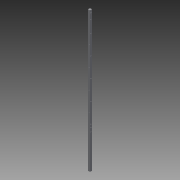
# Autodesk Inventor part: Aluminium Rod
Saved by Autodesk Inventor 2015 (Build 190159000, 159)
## iProperties
Created: 2014-09-22
Part Number: Aluminium Rod
Material: Generic
Document SubType Name: Modeling
Designer: I Rabey
Density: 1 g/cm^3
Appearance: Default
Author: I Rabey
Autodesk Inventor part; units mm, degrees
ref_plane "YZ Plane" through (0, 0, 0) normal (1, 0, 0) x (0, 1, 0)
ref_plane "XZ Plane" through (0, 0, 0) normal (0, 1, 0) x (-1, 0, 0)
ref_plane "XY Plane" through (0, 0, 0) normal (0, 0, 1) x (1, 0, 0)
sketch "Sketch1" plane through (0, 0, 0) normal (0, 1, 0) x (-1, 0, 0)
  line L0 (-6.35, 6.35) -> (6.35, 6.35)
  line L1 (6.35, 6.35) -> (6.35, -6.35)
  line L2 (6.35, -6.35) -> (-6.35, -6.35)
  line L3 (-6.35, -6.35) -> (-6.35, 6.35)
  line L4 (-6.35, 6.35) -> (6.35, -6.35) construction
  line L5 (6.35, 6.35) -> (-6.35, -6.35) construction
  point P0 (0, 0)
  dimension "d0" = 12.7
  dimension "d1" = 12.7
  constraints: 12 end point, 2 midpoint, 2 parallel, 1 horizontal, 1 perpendicular
  measures "d0" distance of L1.end L2.end
  measures "d1" distance of L0.end L1.end
extrude "Extrusion1" add sketch "Sketch1" along normal blind 903
sketch "Sketch3" plane through (6.35, 0, -6.35) normal (1, 0, 0) x (0, 0, -1)
  circle A0 centre (-6.35, 886.5) radius 2.5
  line L0 (-12.7, 903) -> (0, 903) projected
  point P0 (-6.35, 0)
  dimension "d4" = 5
  dimension "d5" = 16.5
  constraints: 1 centre point
  measures "d4" diameter of A0
  measures "d5" distance from line of L0 A0.centre
sketch "Sketch4" plane through (6.35, 0, -6.35) normal (1, 0, 0) x (0, 0, -1)
  circle A0 centre (-6.35, 848.39) radius 2.5
  line L0 (-12.7, 903) -> (0, 903) projected
  point P0 (-6.35, 0)
  dimension "d6" = 5
  dimension "d7" = 54.61
  constraints: 1 centre point
  measures "d6" diameter of A0
  measures "d7" distance from line of L0 A0.centre
sketch "Sketch5" plane through (6.35, 0, -6.35) normal (1, 0, 0) x (0, 0, -1)
  circle A0 centre (-6.35, 772.34) radius 2.5
  line L0 (-12.7, 903) -> (0, 903) projected
  point P0 (-6.35, 0)
  dimension "d8" = 5
  dimension "d9" = 130.66
  constraints: 1 centre point
  measures "d8" diameter of A0
  measures "d9" distance from line of L0 A0.centre
sketch "Sketch6" plane through (6.35, 0, -6.35) normal (1, 0, 0) x (0, 0, -1)
  circle A0 centre (-6.35, 645.34) radius 2.5
  line L0 (-12.7, 903) -> (0, 903) projected
  point P0 (-6.35, 0)
  dimension "d10" = 5
  dimension "d11" = 257.66
  constraints: 1 centre point
  measures "d10" diameter of A0
  measures "d11" distance from line of L0 A0.centre
sketch "Sketch7" plane through (6.35, 0, -6.35) normal (1, 0, 0) x (0, 0, -1)
  circle A0 centre (-6.35, 518.34) radius 2.5
  line L0 (-12.7, 903) -> (0, 903) projected
  point P0 (-6.35, 0)
  dimension "d12" = 5
  dimension "d13" = 384.66
  constraints: 1 centre point
  measures "d12" diameter of A0
  measures "d13" distance from line of L0 A0.centre
sketch "Sketch8" plane through (6.35, 0, -6.35) normal (1, 0, 0) x (0, 0, -1)
  circle A0 centre (-6.35, 391.34) radius 2.5
  line L0 (-12.7, 903) -> (0, 903) projected
  point P0 (-6.35, 0)
  dimension "d14" = 5
  dimension "d15" = 511.66
  constraints: 1 centre point
  measures "d14" diameter of A0
  measures "d15" distance from line of L0 A0.centre
sketch "Sketch9" plane through (6.35, 0, -6.35) normal (1, 0, 0) x (0, 0, -1)
  circle A0 centre (-6.35, 264.34) radius 2.5
  line L0 (-12.7, 903) -> (0, 903) projected
  point P0 (-6.35, 0)
  dimension "d16" = 5
  dimension "d17" = 638.66
  constraints: 1 centre point
  measures "d16" diameter of A0
  measures "d17" distance from line of L0 A0.centre
sketch "Sketch10" plane through (6.35, 0, -6.35) normal (1, 0, 0) x (0, 0, -1)
  circle A0 centre (-6.35, 246.26) radius 2.5
  line L0 (-12.7, 903) -> (0, 903) projected
  point P0 (-6.35, 0)
  dimension "d18" = 5
  dimension "d19" = 656.74
  constraints: 1 centre point
  measures "d18" diameter of A0
  measures "d19" distance from line of L0 A0.centre
sketch "Sketch11" plane through (6.35, 0, -6.35) normal (1, 0, 0) x (0, 0, -1)
  circle A0 centre (-6.35, 220.86) radius 2.5
  line L0 (-12.7, 903) -> (0, 903) projected
  point P0 (-6.35, 0)
  dimension "d20" = 5
  dimension "d21" = 682.14
  constraints: 1 centre point
  measures "d20" diameter of A0
  measures "d21" distance from line of L0 A0.centre
hole "Hole1" at (6.35, 886.5, 0) direction (-1, 0, 0) diameter 5 end through all
hole "Hole2" at (6.35, 848.39, 0) direction (-1, 0, 0) diameter 5 end through all
hole "Hole3" at (6.35, 772.34, 0) direction (-1, 0, 0) diameter 5 end through all
hole "Hole4" at (6.35, 645.34, 0) direction (-1, 0, 0) diameter 5 end through all
hole "Hole5" at (6.35, 518.34, 0) direction (-1, 0, 0) diameter 5 end through all
hole "Hole6" at (6.35, 391.34, 0) direction (-1, 0, 0) diameter 5 end through all
hole "Hole7" at (6.35, 264.34, 0) direction (-1, 0, 0) diameter 5 end through all
hole "Hole8" at (6.35, 246.26, 0) direction (-1, 0, 0) diameter 5 end through all
hole "Hole9" at (6.35, 220.86, 0) direction (-1, 0, 0) diameter 5 end through all
sketch "Sketch21" plane through (6.35, 0, 6.35) normal (0, 0, 1) x (1, 0, 0)
  circle A0 centre (-6.35, 708.84) radius 2.5
  line L0 (-12.7, 903) -> (0, 903) projected
  point P0 (-6.35, 0)
  dimension "d161" = 5
  dimension "d162" = 194.16
  constraints: 1 centre point
  measures "d161" diameter of A0
  measures "d162" distance from line of L0 A0.centre
sketch "Sketch22" plane through (6.35, 0, 6.35) normal (0, 0, 1) x (1, 0, 0)
  circle A0 centre (-6.35, 581.84) radius 2.5
  line L0 (-12.7, 903) -> (0, 903) projected
  point P0 (-6.35, 0)
  dimension "d163" = 5
  dimension "d164" = 321.16
  constraints: 1 centre point
  measures "d163" diameter of A0
  measures "d164" distance from line of A0.centre L0
sketch "Sketch23" plane through (6.35, 0, 6.35) normal (0, 0, 1) x (1, 0, 0)
  circle A0 centre (-6.35, 454.895) radius 2.5
  line L0 (-12.7, 903) -> (0, 903) projected
  point P0 (-6.35, 0)
  dimension "d165" = 5
  dimension "d166" = 448.105
  constraints: 1 centre point
  measures "d165" diameter of A0
  measures "d166" distance from line of L0 A0.centre
sketch "Sketch24" plane through (6.35, 0, 6.35) normal (0, 0, 1) x (1, 0, 0)
  circle A0 centre (-6.35, 327.84) radius 2.5
  line L0 (-12.7, 903) -> (0, 903) projected
  point P0 (-6.35, 0)
  dimension "d167" = 5
  dimension "d168" = 575.16
  constraints: 1 centre point
  measures "d167" diameter of A0
  measures "d168" distance from line of L0 A0.centre
hole "Hole18" at (0, 708.84, 6.35) direction (0, 0, -1) diameter 5 end through all
hole "Hole19" at (0, 581.84, 6.35) direction (0, 0, -1) diameter 5 end through all
hole "Hole20" at (0, 454.895, 6.35) direction (0, 0, -1) diameter 5 end through all
hole "Hole21" at (0, 327.84, 6.35) direction (0, 0, -1) diameter 5 end through all
body "Solid1"
